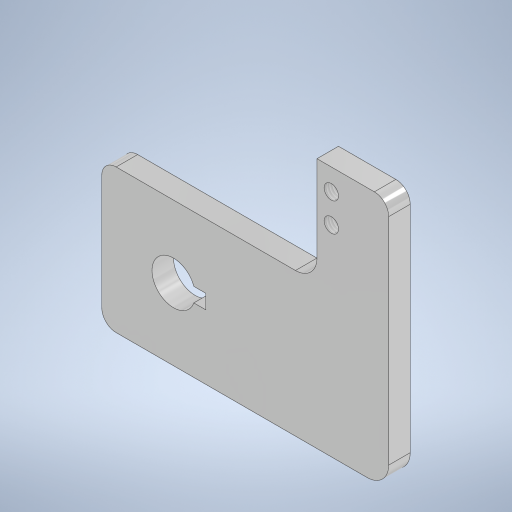
# Autodesk Inventor part: cutter_holder
Saved by Autodesk Inventor 2024 (Build 280153000, 153)
## iProperties
Created: 2025-02-08
Part Number: cutter_holder
Material: アルミニウム 7075
Document SubType Name: Modeling
Designer: 1412z
Density: 2.81 g/cm^3
Appearance: アルミニウム - ダーク
Author: 1412z
Autodesk Inventor part; units mm, degrees
ref_plane "YZ Plane" through (0, 0, 0) normal (1, 0, 0) x (0, 1, 0)
ref_plane "XZ Plane" through (0, 0, 0) normal (0, 1, 0) x (-1, 0, 0)
ref_plane "XY Plane" through (0, 0, 0) normal (0, 0, 1) x (1, 0, 0)
sketch "スケッチ1" plane through (0, 0, 0) normal (0, 0, 1) x (1, 0, 0)
  line L0 (0, 0) -> (0, 20)
  line L1 (0, 0) -> (40, 0)
  line L2 (40, 0) -> (40, 35)
  line L3 (40, 35) -> (30, 35)
  line L4 (30, 35) -> (30, 20)
  line L5 (30, 20) -> (0, 20)
  circle A0 centre (10, 10) radius 3
  line L6 (10, 10) -> (10, 9)
  line L7 (10, 10) -> (10, 11)
  line L8 (10, 9) -> (14.5, 9)
  line L9 (14.5, 9) -> (14.5, 11)
  line L10 (14.5, 11) -> (10, 11)
  point P0 (12.8284, 9)
  point P1 (12.8284, 11)
  dimension "d0" = 20
  dimension "d1" = 40
  dimension "d2" = 35
  dimension "d3" = 10
  dimension "d4" = 6
  dimension "d6" = 1
  dimension "d7" = 1
  dimension "d8" = 4.5
  constraints: 22 end point, 5 perpendicular, 4 vertical, 2 horizontal, 1 centre point
  measures "d0" distance of L0.start L0.end
  measures "d1" distance of L0.start L1.end
  measures "d2" distance of L1.end L2.end
  measures "d3" distance of L2.end L3.end
  measures "d4" diameter of A0
  measures "d6" distance of L6.start L6.end
  measures "d7" distance of L6.start L7.end
  measures "d8" distance of L6.end L8.end
extrude "押し出し1" add sketch "スケッチ1" along normal blind 3
fillet "フィレット1" radius 3 2 edges at (30, 20, 1.5) (40, 0, 1.5)
fillet "フィレット2" radius 2 2 edges at (0, 20, 1.5) (0, 0, 1.5)
fillet "フィレット3" radius 2 1 edges at (40, 35, 1.5)
sketch "スケッチ3" plane through (0, 0, 3) normal (0, 0, 1) x (1, 0, 0)
  circle A0 centre (32, 28) radius 1
  circle A1 centre (32, 32) radius 1
  point P0 (0, 0)
  dimension "d23" = 2
  dimension "d24" = 2
  constraints: 2 centre point
  measures "d23" diameter of A0
  measures "d24" diameter of A1
extrude "押し出し3" cut sketch "スケッチ3" against normal blind 10
thread "ねじ3" size "M2x0.4" class "6H" standard "ANSI Metric M Profile" full length
thread "ねじ4" size "M2x0.4" class "6H" standard "ANSI Metric M Profile" full length
